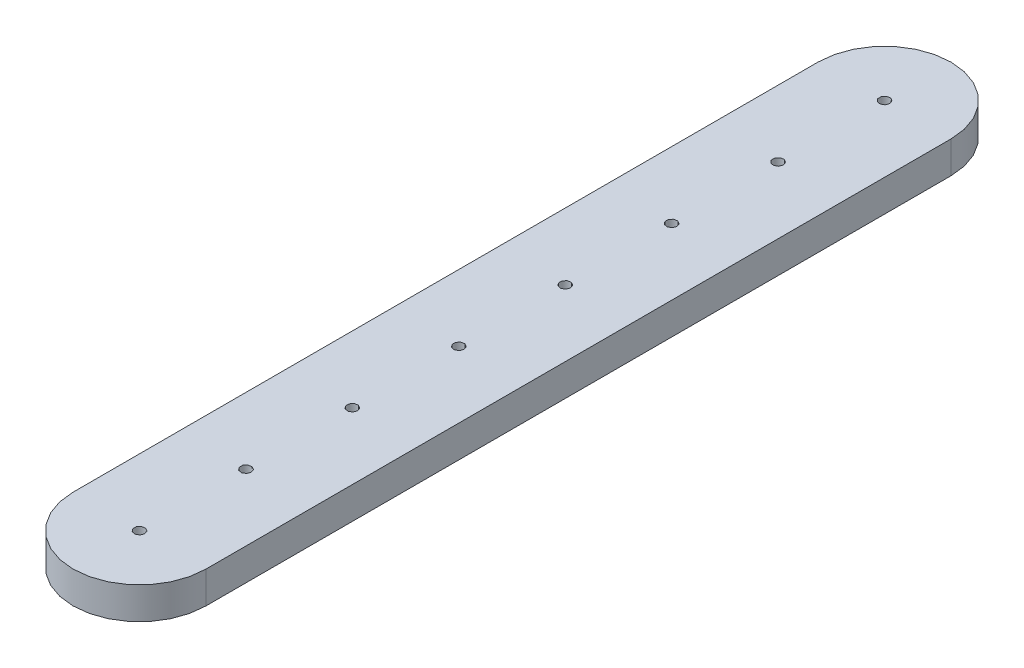
# Autodesk Inventor part: Part6
Saved by Autodesk Inventor 2026.1 (Build 301233020, 233B)
## iProperties
Created: 2026-03-19
Part Number: Part6
Material: Generic
Document SubType Name: Modeling
Designer: Owen L
Density: 1 g/cm^3
Appearance: Default
Author: Owen L
Autodesk Inventor part; units mm, degrees
ref_plane "YZ Plane" through (0, 0, 0) normal (1, 0, 0) x (0, 1, 0)
ref_plane "XZ Plane" through (0, 0, 0) normal (0, 1, 0) x (-1, 0, 0)
ref_plane "XY Plane" through (0, 0, 0) normal (0, 0, 1) x (1, 0, 0)
sketch "Sketch1" plane through (0, 0, 0) normal (0, 1, 0) x (-1, 0, 0)
  line L0 (0, -88.9) -> (0, 88.9) construction
  line L1 (15.875, -88.9) -> (15.875, 88.9)
  line L2 (-15.875, 88.9) -> (-15.875, -88.9)
  arc A0 (-15.875, -88.9) -> (15.875, -88.9) centre (0, -88.9) ccw
  arc A1 (15.875, 88.9) -> (-15.875, 88.9) centre (0, 88.9) ccw
  point P0 (0, 0)
  point P1 (0, 63.5)
  point P2 (0, 38.1)
  point P3 (0, 12.7)
  point P4 (0, -12.7)
  point P5 (0, -38.1)
  point P6 (0, -63.5)
  point P7 (0, -88.9)
  dimension "d0" = 31.75
  dimension "d1" = 177.8
  dimension "d4" = 25.4
  constraints: 8 end point, 4 point on circle, 4 tangent, 2 centre point, 2 vertical, 1 coincident, 1 midpoint, 1 parallel, 7 other
  measures "d0" distance between parallel lines of L1 L2
  measures "d1" distance of L0.start L0.end
  measures "d4" distance of point (0, 88.9) point (0, 63.5)
extrude "Extrusion1" add sketch "Sketch1" along normal blind 7.62
hole "Hole1" at (0, 0, 88.9) at (0, 0, 63.5) at (0, 0, 38.1) at (0, 0, 12.7) at (0, 0, -12.7) at (0, 0, -38.1) at (0, 0, -63.5) at (0, 0, -88.9) direction (0, 1, 0) diameter 2.54 end through all
body "Solid1"
